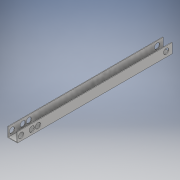
# Autodesk Inventor part: 36in Aluminum Channel
Saved by Autodesk Inventor 2018 (Build 220112000, 112)
## iProperties
Created: 2019-01-15
Part Number: 36in Aluminum Channel
Material: Generic
Document SubType Name: Modeling
Designer: Gabriel
Density: 1 g/cm^3
Appearance: Default
Author: Gabriel
Autodesk Inventor part; units mm, degrees
ref_plane "YZ Plane" through (0, 0, 0) normal (1, 0, 0) x (0, 1, 0)
ref_plane "XZ Plane" through (0, 0, 0) normal (0, 1, 0) x (-1, 0, 0)
ref_plane "XY Plane" through (0, 0, 0) normal (0, 0, 1) x (1, 0, 0)
sketch "Sketch1" plane through (0, 0, 0) normal (0, 1, 0) x (-1, 0, 0)
  line L0 (1.7293, -2.0233) -> (-49.0707, -2.0233)
  line L1 (-49.0707, -2.0233) -> (-49.0707, 810.7767)
  line L2 (-49.0707, 810.7767) -> (1.7293, 810.7767)
  line L3 (1.7293, 810.7767) -> (1.7293, -2.0233)
  point P0 (0, 0)
  dimension "d0" = 50.8
  dimension "d1" = 812.8
  constraints: 8 end point, 2 parallel, 1 horizontal, 1 perpendicular
  measures "d0" distance of L1.end L2.end
  measures "d1" distance of L0.end L1.end
extrude "Extrusion1" add sketch "Sketch1" along normal blind 50.8
sketch "Sketch2" plane through (0, 50.8, 0) normal (0, 1, 0) x (1, 0, 0)
  line L0 (49.0707, 2.0233) -> (-1.7293, 2.0233) projected
  line L1 (-1.7293, 2.0233) -> (1.4457, 2.0233)
  line L2 (49.0707, 2.0233) -> (45.8957, 2.0233)
  line L3 (1.4457, 2.0233) -> (45.8957, 2.0233)
  line L4 (45.8957, 2.0233) -> (45.8957, -810.7767)
  line L5 (45.8957, -810.7767) -> (1.4457, -810.7767)
  line L6 (1.4457, -810.7767) -> (1.4457, 2.0233)
  point P0 (0, 0)
  dimension "d4" = 3.175
  dimension "d5" = 3.175
  dimension "d6" = 44.45
  dimension "d7" = 812.8
  constraints: 12 end point, 2 parallel, 2 point on line, 1 horizontal, 1 perpendicular
  measures "d4" distance of L0.end L1.end
  measures "d5" distance of L0.start L2.end
  measures "d6" distance of L4.end L5.end
  measures "d7" distance of L3.end L4.end
extrude "Extrusion2" cut sketch "Sketch2" against normal blind 47.625
sketch "Sketch3" plane through (49.0707, 0, 810.7767) normal (1, 0, 0) x (0, 0, -1)
  line L0 (0, 0) -> (0, 50.8) projected
  line L1 (0, 25.4) -> (19.05, 25.4)
  circle A0 centre (19.05, 25.4) radius 14.2875
  line L2 (19.05, 25.4) -> (76.2, 25.4)
  circle A1 centre (76.2, 25.4) radius 14.2875
  line L3 (76.2, 25.4) -> (107.95, 25.4)
  circle A2 centre (107.95, 25.4) radius 14.2875
  point P0 (810.7767, 0)
  dimension "d10" = 19.05
  dimension "d11" = 28.575
  dimension "d12" = 57.15
  dimension "d13" = 28.575
  dimension "d14" = 31.75
  dimension "d15" = 28.575
  constraints: 6 end point, 3 centre point, 3 coincident, 3 horizontal, 1 midpoint
  measures "d10" distance of L1.start L1.end
  measures "d11" diameter of A0
  measures "d12" distance of L2.start L2.end
  measures "d13" diameter of A1
  measures "d14" distance of L3.start L3.end
  measures "d15" diameter of A2
extrude "Extrusion3" cut sketch "Sketch3" against normal blind 76.2
sketch "Sketch4" plane through (49.0707, 0, 810.7767) normal (1, 0, 0) x (0, 0, -1)
  line L0 (812.8, 50.8) -> (812.8, 3.175) projected
  line L1 (812.8, 26.9875) -> (781.05, 26.9875)
  circle A0 centre (781.05, 26.9875) radius 14.2875
  point P0 (810.7767, 0)
  dimension "d18" = 31.75
  dimension "d19" = 28.575
  constraints: 2 end point, 1 centre point, 1 coincident, 1 horizontal, 1 midpoint
  measures "d18" distance of L1.start L1.end
  measures "d19" diameter of A0
extrude "Extrusion4" cut sketch "Sketch4" against normal blind 76.2
body "Solid1"
